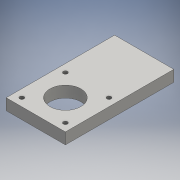
# Autodesk Inventor part: nema17 x plate
Saved by Autodesk Inventor 2016 SP1 (Build 200210100, 210)
## iProperties
Created: 2016-05-25
Part Number: nema17 x plate
Material: Generic
Document SubType Name: Modeling
Designer: ubik
Density: 1 g/cm^3
Appearance: Default
Author: ubik
Autodesk Inventor part; units mm, degrees
ref_plane "YZ Plane" through (0, 0, 0) normal (1, 0, 0) x (0, 1, 0)
ref_plane "XZ Plane" through (0, 0, 0) normal (0, 1, 0) x (-1, 0, 0)
ref_plane "XY Plane" through (0, 0, 0) normal (0, 0, 1) x (1, 0, 0)
sketch "Sketch1" plane through (0, 0, 0) normal (0, 0, 1) x (1, 0, 0)
  circle A0 centre (0, 0) radius 11 projected
  circle A1 centre (-15.5, 15.5) radius 1.5 projected
  circle A2 centre (15.5, 15.5) radius 1.5 projected
  circle A3 centre (-15.5, -15.5) radius 1.5 projected
  circle A4 centre (15.5, -15.5) radius 1.5 projected
  line L0 (21.05, -21.05) -> (-21.05, -21.05)
  line L1 (21.05, 21.05) -> (21.05, -21.05)
  line L2 (-21.05, 21.05) -> (21.05, 21.05)
  line L3 (-21.05, -21.05) -> (-21.05, 21.05)
  point P0 (0, 0)
  constraints: 8 end point
extrude "Extrusion1" add sketch "Sketch1" along normal blind 8
sketch "Sketch2" plane through (-21.05, 21.05, 0) normal (0, 1, 0) x (1, 0, 0)
  line L0 (42.1, 0) -> (0, 0) projected
  line L1 (0, 0) -> (0, -8) projected
  line L2 (42.1, -8) -> (0, -8) projected
  line L3 (42.1, 0) -> (42.1, -8) projected
  point P0 (21.05, 0)
extrude "Extrusion2" add sketch "Sketch2" along normal blind 35
body "Solid1"
